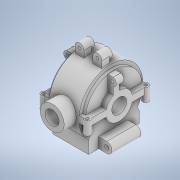
# Autodesk Inventor part: PX9200-13
Saved by Autodesk Inventor 2022.3 (Build 263350000, 350)
## iProperties
Created: 2022-07-21
Part Number: PX9200-13
Material: Generic
Document SubType Name: Modeling
Designer: luis_
Density: 1 g/cm^3
Appearance: Default
Author: luis_
Autodesk Inventor part; units mm, degrees
ref_plane "YZ Plane" through (0, 0, 0) normal (1, 0, 0) x (0, 1, 0)
ref_plane "XZ Plane" through (0, 0, 0) normal (0, 1, 0) x (-1, 0, 0)
ref_plane "XY Plane" through (0, 0, 0) normal (0, 0, 1) x (1, 0, 0)
sketch "Sketch1" plane through (0, 0, 0) normal (1, 0, 0) x (0, 1, 0)
  arc A0 (-12.938383, -16.982955) -> (-12.938383, 16.982955) centre (0, 0) ccw
  circle A1 centre (0, 0) radius 5
  line L0 (-21.606091, 16.982955) -> (-12.938383, 16.982955)
  line L1 (-12.938383, -16.982955) -> (-21.606091, -16.982955)
  line L2 (-21.606091, 16.982955) -> (-21.606091, -16.982955)
  line L3 (-21.606091, 10.217045) -> (-14.606091, 10.217045)
  line L4 (-14.606091, 10.217045) -> (-14.606091, -9.182955)
  line L5 (-14.606091, -9.182955) -> (-21.606091, -9.182955)
  circle A2 centre (0, 0) radius 9
  line L6 (2.2, 22) -> (-2.2, 22)
  line L7 (-2.2, 22) -> (-2.2, 8.72697)
  line L8 (2.2, 8.72697) -> (2.2, 22)
  line L9 (0.756177, -19.72697) -> (-0.804929, -19.72697)
  line L10 (0.756177, -19.72697) -> (2.2, -19.72697)
  line L11 (-0.804929, -19.72697) -> (-2.2, -19.72697)
  line L12 (2.2, -22) -> (2.124404, -21.244044) construction
  line L13 (2.2, -19.72697) -> (2.2, -8.72697)
  line L14 (-2.2, -8.72697) -> (-2.2, -19.72697)
  arc A3 (-10.606091, -15.764226) -> (-10.606091, 15.764226) centre (0, 0) ccw
  line L15 (-10.606091, -15.764226) -> (-12.938383, -16.982955)
  line L16 (-12.938383, 16.982955) -> (-10.606091, 15.764226)
  line L17 (9, 0) -> (18.574176, 0)
  line L18 (18.574176, 0) -> (18.574176, 4)
  line L19 (18.574176, 4) -> (9, 4)
  line L20 (9, 4) -> (8.062258, 4)
  line L21 (19, 0) -> (27.35, 0)
  line L22 (27.35, 0) -> (27.35, 5)
  line L23 (27.35, 5) -> (20.756264, 5)
  point P0 (-21.606091, 0)
  point P1 (-0.024376, -19.72697)
  point P2 (21.35, 0)
  point P3 (-10.606091, 15.764226)
  point P4 (-2.2, -18.872202)
  point P5 (-2.2, 18.872202)
  point P6 (2.2, -18.872202)
  point P7 (2.2, 18.872202)
  point P8 (-2.2, 21.236349)
  point P9 (2.2, 21.236349)
  point P10 (21.35, 0)
  dimension "d0" = 42.7
  dimension "d1" = 10
  dimension "d6" = 19.4
  dimension "d7" = 18
  dimension "d8" = 4.4
  dimension "d14" = 38
  constraints: 48 end point, 15 point on circle, 8 parallel, 6 horizontal, 4 centre point, 4 coincident, 4 perpendicular, 3 point on line, 2 midpoint
  measures "d0" diameter of A0
  measures "d1" diameter of A1
  measures "d6" distance of L3.end L4.end
  measures "d7" diameter of A2
  measures "d8" distance of L6.end L6.start
  measures "d14" diameter of A3
extrude "Extrusion1" add sketch "Sketch1" along normal mid plane 24 contours L1 L2 L5 L4 L3 L0 L16 A3 L7 A2 L14 L15 | A3 L13 A2 L17 L18 | L19 L20 A2 L8 A3
extrude "Extrusion2" add sketch "Sketch1" along normal mid plane 20 contours L15 A3 L14 L11 L9 L10 L13 L21 A0 | L21 A3 L8 A0 | L7 A3 L16 A0
extrude "Extrusion3" add sketch "Sketch1" along normal mid plane 31.2 contours A3 L13 L10 L9 L11 L14 | L14 A2 L13 A3 | L8 A3 L7 A0 | L18 L17 A2 L20 L19 | A2 | L8 A2 L7 A3
extrude "Extrusion4" add sketch "Sketch1" along normal mid plane 18 contours A0 L23 L22 L21
extrude "Extrusion5" add sketch "Sketch1" along normal mid plane 42 contours L2 L3 L4 L5
sketch "Sketch2" plane through (0, 0, 0) normal (1, 0, 0) x (0, 1, 0)
  arc A0 (-12.938383, -16.982955) -> (2.2, 21.236349) centre (0, 0) ccw
  line L0 (21.35, -0.000064) -> (27.35, -0.000064)
  line L1 (27.35, 0) -> (27.35, 5)
  line L2 (27.35, -0.000064) -> (27.35, 5)
  line L3 (27.35, 5) -> (20.756264, 5)
  line L4 (27.35, 5) -> (20.756264, 5)
  arc A1 (21.35, -0.000064) -> (20.756264, 5) centre (0, 0) ccw
  constraints: 6 end point, 3 point on circle, 2 collinear, 1 centre point, 1 concentric, 1 horizontal
extrude "Extrusion6" cut sketch "Sketch2" along normal mid plane 6
sketch "Sketch3" plane through (-15.6, 18.574176, 4) normal (0, 0, 1) x (1, 0, 0)
  arc A0 (0.6, 0) -> (0, -5.332489) centre (0.6, -2.7) ccw
  line L0 (0, 0) -> (3.6, 0)
  line L1 (3.6, 0) -> (3.6, -16.374176)
  arc A1 (31.2, -5.332492) -> (31.2, -0.067508) centre (30.600012, -2.7) ccw
  line L2 (27.6, 0) -> (31.2, 0)
  line L3 (0, -10.511918) -> (0, 0)
  line L4 (0, -0.067511) -> (0, 0)
  line L5 (31.2, -9.574176) -> (31.2, 0)
  circle A2 centre (30.600012, -2.7) radius 0.5
  circle A3 centre (0.6, -2.7) radius 0.5
  point P0 (15.6, -18.574176)
  dimension "d32" = 5.4
  dimension "d33" = 3
  dimension "d34" = 5.4
  dimension "d35" = 1
  dimension "d36" = 1
  constraints: 5 point on circle, 4 centre point, 4 point on line, 2 coincident, 2 end point, 2 tangent, 1 collinear
  measures "d32" diameter of A0
  measures "d33" distance from line of L1 A0.centre
  measures "d34" diameter of A1
  measures "d35" diameter of A2
  measures "d36" diameter of A3
extrude "Extrusion7" add sketch "Sketch3" against normal blind 5 contours L3 A0 | L5 A1
sketch "Sketch4" plane through (-12, 9, 0) normal (0, 0, -1) x (-1, 0, 0)
  line L0 (3.6, 9.574176) -> (0, 9.574176)
  line L1 (3.6, 9.506665) -> (3.6, 4.241686)
  line L2 (0, 9.574176) -> (3.6, 9.574176)
  line L3 (3.6, 9.574176) -> (3.6, 4.241686)
  line L4 (3.6, 4.241686) -> (0, 4.241686)
  line L5 (0, 4.241686) -> (0, 9.574176)
  line L6 (-24, 9.574176) -> (-27.6, 9.574176)
  line L7 (-27.6, 9.574176) -> (-24, 9.574176)
  line L8 (-24, 9.574176) -> (-24, 4.241686)
  line L9 (-24, 4.241686) -> (-27.6, 4.241686)
  line L10 (-27.6, 4.241686) -> (-27.6, 9.574176)
  point P0 (-12, -9)
  point P1 (3.6, 9.506665)
  point P2 (3.6, 9.574176)
  constraints: 16 end point, 4 parallel, 2 horizontal, 2 perpendicular, 1 point on line
extrude "Extrusion8" add sketch "Sketch4" along normal blind 1
sketch "Sketch5" plane through (-15.6, 18.574176, -1) normal (0, 0, -1) x (-1, 0, 0)
  arc A0 (0, -5.332489) -> (0, -0.067511) centre (-0.6, -2.7) ccw
  circle A1 centre (-0.6, -2.7) radius 1
  arc A2 (-31.2, -0.067508) -> (-31.2, -5.332492) centre (-30.600012, -2.7) ccw
  circle A3 centre (-30.600012, -2.7) radius 1
  point P0 (-15.6, -18.574176)
  dimension "d41" = 2
  dimension "d42" = 2
  constraints: 2 centre point, 2 coincident
  measures "d41" diameter of A1
  measures "d42" diameter of A3
extrude "Extrusion9" cut sketch "Sketch5" against normal blind 5
sketch "Sketch6" plane through (9, 21.35, 0) normal (0, 0, -1) x (-1, 0, 0)
  line L0 (6, 0) -> (0, 0)
  line L1 (18, 0) -> (12, 0)
  circle A0 centre (3, 4) radius 3
  circle A1 centre (15, 4) radius 3
  line L2 (6, 6) -> (0, 6)
  line L3 (0.763932, 6) -> (5.236068, 6)
  line L4 (12, 6) -> (18, 6)
  line L5 (12.763932, 6) -> (17.236068, 6)
  line L6 (0, 0) -> (0, 6)
  line L7 (0, 4) -> (0, 6)
  line L8 (0, 6) -> (0.763932, 6)
  line L9 (5.236068, 6) -> (6, 6)
  line L10 (12, -0.593736) -> (12, 6)
  line L11 (12, 4) -> (12, 6)
  line L12 (12, 6) -> (12.763932, 6)
  line L13 (18, 6) -> (18, 0)
  line L14 (17.236068, 6) -> (18, 6)
  line L15 (18, 6) -> (18, 4)
  arc A2 (18, 4) -> (17.236068, 6) centre (15, 4) ccw
  arc A3 (12.763932, 6) -> (12, 4) centre (15, 4) ccw
  line L16 (6, 0) -> (6, 6)
  arc A4 (6, 4) -> (5.236068, 6) centre (3, 4) ccw
  arc A5 (0.763932, 6) -> (0, 4) centre (3, 4) ccw
  point P0 (9, -21.35)
  point P1 (3, 0)
  point P2 (15, 0)
  dimension "d45" = 4
  dimension "d46" = 4
  constraints: 18 end point, 18 point on circle, 8 point on line, 6 centre point, 4 collinear, 4 concentric, 2 coincident, 2 midpoint, 2 tangent, 1 horizontal, 1 vertical
  measures "d45" distance of point (3, 0) point (3, 4)
  measures "d46" distance of point (15, 0) point (15, 4)
extrude "Extrusion10" add sketch "Sketch6" along normal blind 2 contours A0 L2 | L2 A0 | A1 L4 | L4 A1
extrude "Extrusion11" add sketch "Sketch6" against normal blind 5 contours L2 A0 | L4 A1 picked at (2.434728, 6.158238) picked at (15.565272, 6.158238)
extrude "Extrusion12" cut sketch "Sketch6" against normal blind 5 contours A0 L2 L16 | L6 L2 A0 | A1 L4 L13 | L10 L4 A1
sketch "Sketch7" plane through (6, 25.35, -2) normal (0, 0, -1) x (-1, 0, 0)
  circle A0 centre (0, 0) radius 1
  circle A1 centre (12, 0) radius 3 projected
  circle A2 centre (12, 0) radius 1
  point P0 (6, -25.35)
  dimension "d53" = 2
  dimension "d54" = 2
  constraints: 2 centre point, 1 coincident
  measures "d53" diameter of A0
  measures "d54" diameter of A2
extrude "Extrusion13" cut sketch "Sketch7" against normal blind 1000 contours A0 | A2
sketch "Sketch8" plane through (-15.6, -2.2, 21.236349) normal (0, -1, 0) x (1, 0, 0)
  circle A0 centre (1, -1) radius 2
  line L0 (0, -12.509379) -> (0, 0)
  line L1 (0, 0) -> (5.6, 0)
  circle A1 centre (1, -39.963318) radius 2
  circle A2 centre (30.2, -39.963318) radius 2
  circle A3 centre (30.2, -1) radius 2
  line L2 (0, -40.963318) -> (0, -29.963318)
  line L3 (0, -40.963318) -> (5.6, -40.963318)
  line L4 (31.2, -29.963318) -> (31.2, -40.963318)
  line L5 (25.6, -40.963318) -> (31.2, -40.963318)
  line L6 (31.2, 0) -> (31.2, -12.509379)
  line L7 (25.6, 0) -> (31.2, 0)
  line L8 (31.2, -2.732051) -> (31.2, 0.097617)
  line L9 (31.2, 0.097617) -> (28.538741, 0.113651)
  line L10 (0, 0.113651) -> (31.2, 0.113651)
  line L11 (25.6, -40.963318) -> (31.2, -40.963318)
  line L12 (28.467949, -40.963318) -> (31.2, -40.963318)
  line L13 (31.2, -40.963318) -> (31.2, -38.231267)
  line L14 (0, -40.963318) -> (5.6, -40.963318)
  line L15 (2.732051, -40.963318) -> (0, -40.963318)
  line L16 (0, -40.963318) -> (0, -38.231267)
  line L17 (0, -2.732051) -> (0, 0.113651)
  line L18 (2.661259, 0.113651) -> (0, 0.113651)
  circle A4 centre (1, -1) radius 1
  circle A5 centre (1, -39.963318) radius 1
  circle A6 centre (30.2, -39.963318) radius 1
  circle A7 centre (30.2, -1) radius 1
  point P0 (15.6, -21.236349)
  point P1 (2.732051, -40.963318)
  point P2 (28.467949, -40.963318)
  dimension "d57" = 4
  dimension "d58" = 1
  dimension "d59" = 1
  dimension "d60" = 4
  dimension "d61" = 4
  dimension "d62" = 4
  dimension "d63" = 1
  dimension "d64" = 1
  dimension "d65" = 1
  dimension "d66" = 1
  dimension "d67" = 1
  dimension "d68" = 1
  dimension "d69" = 2
  dimension "d70" = 2
  dimension "d71" = 2
  dimension "d72" = 2
  constraints: 16 end point, 8 centre point, 8 point on circle, 8 point on line, 4 coincident, 3 collinear, 1 perpendicular, 1 vertical
  measures "d57" diameter of A0
  measures "d58" distance from line of L0 A0.centre
  measures "d59" distance from line of A0.centre L1
  measures "d60" diameter of A1
  measures "d61" diameter of A2
  measures "d62" diameter of A3
  measures "d63" distance from line of L2 A1.centre
  measures "d64" distance from line of A1.centre L3
  measures "d65" distance from line of A2.centre L4
  measures "d66" distance from line of A2.centre L5
  measures "d67" distance from line of L6 A3.centre
  measures "d68" distance from line of L7 A3.centre
  measures "d69" diameter of A4
  measures "d70" diameter of A5
  measures "d71" diameter of A6
  measures "d72" diameter of A7
extrude "Extrusion14" add sketch "Sketch8" along normal blind 4.4
extrude "Extrusion15" add sketch "Sketch8" against normal blind 4.4 contours L10 L17 L0 A0 | L2 L3 A1 | A2 L5 L4 | A3 L6 L8 L9
extrude "Extrusion16" cut sketch "Sketch8" along normal mid plane 10 contours A4 | A5 | A6 | A7
sketch "Sketch11" plane through (-12, -21.606091, -16.982955) normal (0, -1, 0) x (1, 0, 0)
  line L0 (0, 0) -> (24, 0) projected
  line L1 (-9, 7.8) -> (0, 7.8) projected
  line L2 (24, 0) -> (0, 0)
  line L3 (0, 0) -> (0, 7.8)
  line L4 (0, 7.8) -> (24, 7.8)
  line L5 (24, 7.8) -> (24, 0)
  point P0 (12, 16.982955)
  constraints: 8 end point, 2 parallel, 1 horizontal, 1 perpendicular
extrude "Extrusion17" cut sketch "Sketch11" against normal blind 1
sketch "Sketch12" plane through (-12, -21.606091, 16.982955) normal (0, -1, 0) x (1, 0, 0)
  line L0 (-9, -26.165909) -> (33, -26.165909)
  line L1 (0, 0) -> (24, 0)
  line L2 (0, -6.765909) -> (0, 0)
  line L3 (24, 0) -> (24, -6.765909)
  line L4 (0, -33.965909) -> (0, -26.165909)
  line L5 (24, -26.165909) -> (24, -33.965909)
  circle A0 centre (21, -29.665909) radius 1
  circle A1 centre (3, -29.665909) radius 1
  circle A2 centre (3, -3.5) radius 1
  circle A3 centre (21, -3.5) radius 1
  point P0 (12, -16.982955)
  point P1 (0, -3.382955)
  dimension "d81" = 3.5
  dimension "d82" = 3.5
  dimension "d83" = 3.5
  dimension "d84" = 3.5
  dimension "d85" = 3
  dimension "d86" = 3
  dimension "d87" = 3
  dimension "d88" = 3
  dimension "d89" = 2
  dimension "d90" = 2
  dimension "d91" = 2
  dimension "d92" = 2
  constraints: 4 centre point, 4 coincident, 1 midpoint
  measures "d81" distance from line of point (21, -29.666) L0
  measures "d82" distance from line of L0 point (3, -29.666)
  measures "d83" distance from line of point (3, -3.5) L1
  measures "d84" distance from line of L1 point (21, -3.5)
  measures "d85" horizontal distance of point (0, -3.383) point (3, -3.5)
  measures "d86" distance from line of L3 point (21, -3.5)
  measures "d87" distance from line of point (3, -29.666) L4
  measures "d88" distance from line of L5 point (21, -29.666)
  measures "d89" diameter of A0
  measures "d90" diameter of A1
  measures "d91" diameter of A2
  measures "d92" diameter of A3
extrude "Extrusion18" cut sketch "Sketch12" against normal blind 1
extrude "Extrusion19" cut sketch "Sketch12" against normal blind 3 contours A0 | A1
sketch "Sketch13" plane through (-21, -14.606091, 10.217045) normal (0, 0, 1) x (1, 0, 0)
  line L0 (9, -7) -> (9, 1.667708)
  line L1 (33, 1.667708) -> (33, -7)
  line L2 (0, -7) -> (9, -7)
  circle A0 centre (38.5, -3.5) radius 3.5
  line L3 (42, 0) -> (42, -7)
  circle A1 centre (3.5, -3.5) radius 3.5
  line L4 (0, -7) -> (0, 0)
  circle A2 centre (3.5, -3.5) radius 1.5
  circle A3 centre (38.5, -3.5) radius 1.5
  line L5 (42, 0) -> (33, 0)
  line L6 (38.5, 0) -> (42, 0)
  line L7 (42, 0) -> (42, -7)
  line L8 (33, -7) -> (42, -7)
  arc A4 (38.5, -7) -> (38.5, 0) centre (38.5, -3.5) ccw
  arc A5 (3.5, 0) -> (3.5, -7) centre (3.5, -3.5) ccw
  line L9 (9, 0) -> (0, 0)
  line L10 (3.5, 0) -> (0, 0)
  line L11 (0, 0) -> (0, -7)
  line L12 (0, -7) -> (3.5, -7)
  point P0 (21, 14.606091)
  point P1 (42, -3.5)
  point P2 (0, -3.5)
  dimension "d100" = 7
  dimension "d101" = 7
  dimension "d102" = 3
  dimension "d103" = 3
  constraints: 10 end point, 8 point on circle, 6 centre point, 6 tangent, 3 point on line, 2 coincident, 2 collinear, 2 perpendicular, 1 horizontal
  measures "d100" diameter of A0
  measures "d101" diameter of A1
  measures "d102" diameter of A2
  measures "d103" diameter of A3
extrude "Extrusion20" cut sketch "Sketch13" against normal blind 20 contours L2 L4 A1 | A1 L4 L9 | L5 L3 A0 | A0 L3 L8 | A2 | A3
sketch "Sketch16" plane through (-12.938741, 0, 21.35) normal (0, 0, -1) x (-1, 0, 0)
  circle A0 centre (-12.938741, 0) radius 8
  dimension "d107" = 16
  constraints: 1 centre point, 1 coincident
  measures "d107" diameter of A0
extrude "Extrusion21" add sketch "Sketch16" along normal blind 1.5 and the other way blind 8
sketch "Sketch17" plane through (0, 0, 29.35) normal (0, 0, 1) x (1, 0, 0)
  circle A0 centre (0, 0) radius 4.7
  dimension "d112" = 9.4
  constraints: 1 centre point, 1 coincident
  measures "d112" diameter of A0
extrude "Extrusion22" cut sketch "Sketch17" against normal blind 6.75
body "Solid1"
